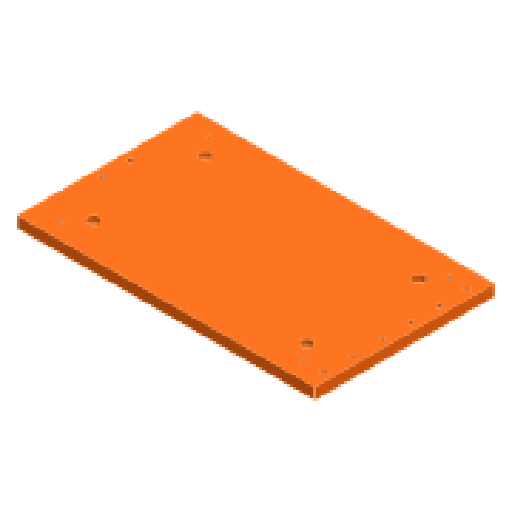
# Autodesk Inventor part: GRJ-03-113
Saved by Autodesk Inventor 2026.1 (Build 301233000, 233)
## iProperties
Company: Gree
Created: 2025-08-20
Part Number: GRJ-03-113
Checked By: Antonio Lucas
Engr Approved By: Antonio Lucas
Material: Fenolite OR
Document SubType Name: Modeling
Mfg Approved By: Anderson Oliveira
Designer: Willian Pinheiro
Mass: 578.125 g
Surface Area: 957.369 cm^2
Volume: 418.931 cm^3
Density: 1.38 g/cm^3
Appearance: Suave - Laranja claro
Description: Base Soldagem
Project: GRJ-03
Dimensões: 10 x 160 x 265 mm
Total: 1
Author: Willian Pinheiro
Revision Number: 00
Title: Soldagem
Autodesk Inventor part; units mm, degrees
ref_plane "YZ Plane" through (0, 0, 0) normal (1, 0, 0) x (0, 1, 0)
ref_plane "XZ Plane" through (0, 0, 0) normal (0, 1, 0) x (-1, 0, 0)
ref_plane "XY Plane" through (0, 0, 0) normal (0, 0, 1) x (1, 0, 0)
sketch "Esboço1" plane through (0, 0, 0) normal (0, 0, 1) x (1, 0, 0)
  line L0 (-185.5, 0) -> (185.5, 0) construction
  line L1 (0, -112) -> (0, 112) construction
  line L2 (-132.5, 80) -> (132.5, 80)
  line L3 (132.5, 80) -> (132.5, -80)
  line L4 (132.5, -80) -> (-132.5, -80)
  line L5 (-132.5, -80) -> (-132.5, 80)
  line L6 (-125, 80) -> (-125, -80) construction
  line L7 (125, 80) -> (125, -80) construction
  line L8 (125, 12.5) -> (125, -12.5) construction
  line L9 (125, 62.64) -> (125, 37.64) construction
  line L10 (125, 12.5) -> (125, -12.5) construction
  line L11 (125, -64.333) -> (125, -39.333) construction
  circle A0 centre (-107.5, -65) radius 10
  circle A1 centre (107.5, -65) radius 10
  circle A2 centre (-107.5, 65) radius 10
  circle A3 centre (107.5, 65) radius 10
  point P0 (0, 0)
  point P1 (-125, 12.5)
  point P2 (-125, -12.5)
  point P3 (125, 0)
  point P4 (125, 50.14)
  point P5 (125, -51.833)
  point P6 (125, 0)
  point P7 (-95, -50)
  point P8 (-95, 50)
  point P9 (95, -50)
  point P10 (95, 50)
  dimension "d0" = 265
  dimension "d1" = 160
  dimension "d3" = 25
  dimension "d5" = 250
  dimension "d6" = 50.14
  dimension "d16" = 51.833
  dimension "d18" = 20
  dimension "d19" = 25
  dimension "d20" = 15
  dimension "d28" = 100
  dimension "d29" = 190
  constraints: 20 end point, 11 symmetric about line, 7 point on line, 4 centre point, 4 midpoint, 3 vertical, 2 collinear, 2 parallel, 1 horizontal, 1 perpendicular, 5 other
  measures "d0" distance of L3.end L4.end
  measures "d1" distance between parallel lines of L2 L4
  measures "d3" distance of L8.end L8.start
  measures "d5" distance between parallel lines of L7 L6
  measures "d6" distance of point (125, 0) point (125, 50.14)
  measures "d16" distance of point (125, -51.833) point (125, 0)
  measures "d18" diameter of A0
  measures "d19" distance from line of L5 A0.centre
  measures "d20" distance from line of L4 A0.centre
  measures "d28" distance of point (-95, 50) point (-95, -50)
  measures "d29" distance of point (95, -50) point (-95, -50)
extrude "Extrusão1" add sketch "Esboço1" along normal blind 10 contours L2 L3 L4 L5 | A0 | A1 | A2 | A3
hole "Furo1" at (-125, 12.5, 0) at (-125, -12.5, 0) at (125, -12.5, 0) at (125, 12.5, 0) at (125, 37.64, 0) at (125, 62.64, 0) at (125, -64.333, 0) at (125, -39.333, 0) direction (0, 0, 1) diameter 4.5 end through all counterbore diameter 8 counterbore depth 4.6 clearance for "Socket Head Cap Screw ISO 4762" size "M4" standard "ISO"
hole "Furo2" at (-107.5, -65, 0) at (107.5, -65, 0) at (107.5, 65, 0) at (-107.5, 65, 0) direction (0, 0, 1) diameter 3.242 end through all thread size "M4x0.7" class "6H" standard "ISO Metric profile"
sketch "Esboço2" plane through (0, 0, 10) normal (0, 0, 1) x (1, 0, 0)
  point P0 (0, 0)
  point P1 (-95, -50)
  point P2 (-95, 50)
  point P3 (95, -50)
  point P4 (95, 50)
hole "Furo3" at (-95, -50, 10) at (-95, 50, 10) at (95, -50, 10) at (95, 50, 10) direction (0, 0, -1) diameter 5.5 end through all counterbore diameter 10 counterbore depth 5.7 clearance for "Socket Head Cap Screw ISO 4762" size "M5" standard "ISO"
fillet "Arredondamento1" radius 0.5 4 edges at (-132.5, -80, 5) (-132.5, 80, 5) (132.5, 80, 5) (132.5, -80, 5)
